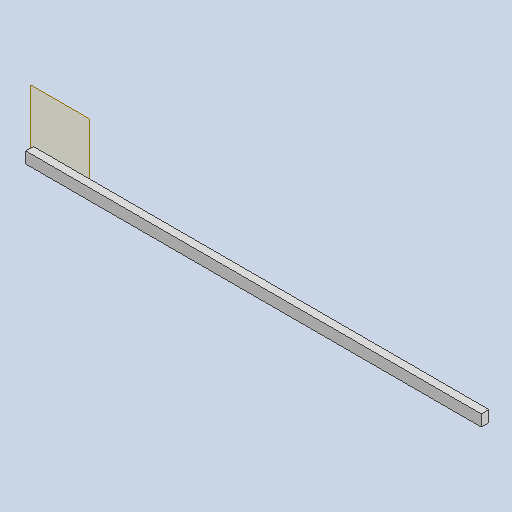
# Autodesk Inventor part: szynka
Saved by Autodesk Inventor 2025 (Build 290162000, 162)
## iProperties
Created: 2025-02-06
Part Number: szynka
Material: Generic
Document SubType Name: Modeling
Designer: piotr
Density: 1 g/cm^3
Appearance: Default
Author: piotr
Autodesk Inventor part; units mm, degrees
ref_plane "YZ Plane" through (0, 0, 0) normal (1, 0, 0) x (0, 1, 0)
ref_plane "XZ Plane" through (0, 0, 0) normal (0, 1, 0) x (-1, 0, 0)
ref_plane "XY Plane" through (0, 0, 0) normal (0, 0, 1) x (1, 0, 0)
ref_plane "Work Plane1" through (0, 0, 0) normal (0, 0, 1) x (1, 0, 0)
sketch "Sketch1" plane through (0, 0, 0) normal (0, 0, 1) x (1, 0, 0)
  line L0 (-35, 35) -> (-35, -35) projected
  line L1 (-35, -35) -> (35, -35) projected
  line L2 (35, -35) -> (35, -30) projected
  line L3 (35, -30) -> (-25, -30) projected
  line L4 (-25, -30) -> (-25, 30) projected
  line L5 (-25, 30) -> (35, 30) projected
  line L6 (35, 30) -> (35, 35) projected
  line L7 (35, 35) -> (-35, 35) projected
  line L8 (-35, -30) -> (565, -30)
  line L9 (565, -30) -> (565, -45)
  line L10 (565, -45) -> (-35, -45)
  line L11 (-35, -45) -> (-35, -30)
  point P0 (0, 0)
  dimension "d0" = 600
  dimension "d1" = 15
  constraints: 8 end point, 2 parallel, 1 horizontal, 1 perpendicular, 1 point on line
  measures "d0" distance of L9.end L10.end
  measures "d1" distance of L8.end L9.end
extrude "Extrusion1" add sketch "Sketch1" along normal blind 10 contours L8 L3 L2 L1 L0 | L1 L2 L8 L9 L10 L11
body "Solid1"
